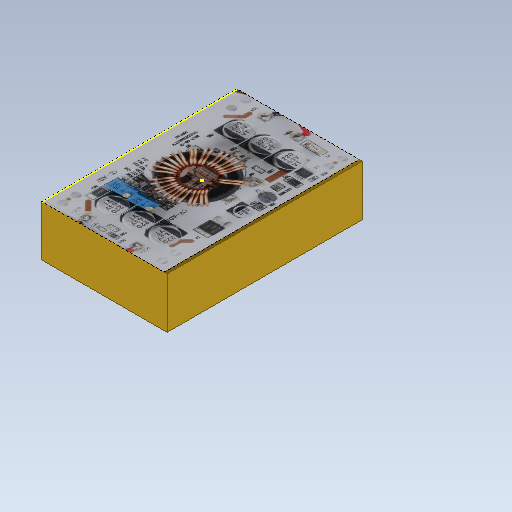
# Autodesk Inventor part: SN-A1401220
Saved by Autodesk Inventor 2020 (Build 240168000, 168)
## iProperties
Created: 2024-09-19
Part Number: SN-A1401220
Material: Типовые
Document SubType Name: Modeling
Designer: Ivan
Density: 1 g/cm^3
Appearance: Фольга — золотистая
Author: Ivan
Autodesk Inventor part; units mm, degrees
ref_plane "YZ Plane" through (0, 0, 0) normal (1, 0, 0) x (0, 1, 0)
ref_plane "XZ Plane" through (0, 0, 0) normal (0, 1, 0) x (-1, 0, 0)
ref_plane "XY Plane" through (0, 0, 0) normal (0, 0, 1) x (1, 0, 0)
sketch "Эскиз1" plane through (0, 0, 0) normal (0, 1, 0) x (-1, 0, 0)
  line L0 (26, 40.5) -> (-26, 40.5)
  line L1 (-26, 40.5) -> (-26, -40.5)
  line L2 (-26, -40.5) -> (26, -40.5)
  line L3 (26, -40.5) -> (26, 40.5)
  line L4 (26, 40.5) -> (-26, -40.5) construction
  point P0 (0, 0)
  point P1 (0, 0)
  dimension "d0" = 52
  dimension "d1" = 81
  constraints: 10 end point, 2 parallel, 1 coincident, 1 horizontal, 1 midpoint, 1 perpendicular
  measures "d0" distance of L2.end L1.end
  measures "d1" distance of L1.end L0.end
extrude "Выдавливание1" add sketch "Эскиз1" along normal blind 21
sketch "Эскиз2" plane through (0, 21, 0) normal (0, 1, 0) x (1, 0, 0)
  line L0 (-26, 40.5) -> (-26, -40.5) projected
  line L1 (-26, -40.5) -> (-26, 40.5) construction
  line L2 (-26, 40.5) -> (24.7494, 40.5) construction
  line L3 (24.7494, 40.5) -> (24.7494, -40.5) construction
  line L4 (24.7494, -40.5) -> (-26, -40.5) construction
  point P0 (0, 0)
  constraints: 1 coincident, 2 other
